Autodesk Inventor part; units mm, degrees
(part 3 of 4)
  line L1419 (-51.1011, -48.3705) -> (-50.3814, -49.0902) construction
  line L1420 (-50.3814, -49.0902) -> (-50.3814, -49.9795) construction
  spline S136 degree 3 poles (-46.3996, -18.0009) (-46.3996, -18.8902) (-47.1193, -19.6113) (-48.0086, -19.6113) knots 0 0 0 0 1 1 1 1
  line L1421 (-46.3996, -18.0009) -> (-46.3996, -18.8902) construction
  line L1422 (-46.3996, -18.8902) -> (-47.1193, -19.6113) construction
  line L1423 (-47.1193, -19.6113) -> (-48.0086, -19.6113) construction
  spline S137 degree 3 poles (-48.0086, -19.6113) (-48.8993, -19.6113) (-49.619, -18.8902) (-49.619, -18.0009) knots 0 0 0 0 1 1 1 1
  line L1424 (-48.0086, -19.6113) -> (-48.8993, -19.6113) construction
  line L1425 (-48.8993, -19.6113) -> (-49.619, -18.8902) construction
  line L1426 (-49.619, -18.8902) -> (-49.619, -18.0009) construction
  spline S138 degree 3 poles (-49.619, -18.0009) (-49.619, -17.1116) (-48.8993, -16.3919) (-48.0086, -16.3919) knots 0 0 0 0 1 1 1 1
  line L1427 (-49.619, -18.0009) -> (-49.619, -17.1116) construction
  line L1428 (-49.619, -17.1116) -> (-48.8993, -16.3919) construction
  line L1429 (-48.8993, -16.3919) -> (-48.0086, -16.3919) construction
  spline S139 degree 3 poles (-48.0086, -16.3919) (-47.1193, -16.3919) (-46.3996, -17.1116) (-46.3996, -18.0009) knots 0 0 0 0 1 1 1 1
  line L1430 (-48.0086, -16.3919) -> (-47.1193, -16.3919) construction
  line L1431 (-47.1193, -16.3919) -> (-46.3996, -17.1116) construction
  line L1432 (-46.3996, -17.1116) -> (-46.3996, -18.0009) construction
  spline S140 degree 3 poles (-72.7019, -7.3708) (-72.7019, -8.0905) (-73.2534, -8.6406) (-73.9731, -8.6406) knots 0 0 0 0 1 1 1 1
  line L1433 (-72.7019, -7.3708) -> (-72.7019, -8.0905) construction
  line L1434 (-72.7019, -8.0905) -> (-73.2534, -8.6406) construction
  line L1435 (-73.2534, -8.6406) -> (-73.9731, -8.6406) construction
  spline S141 degree 3 poles (-73.9731, -8.6406) (-74.6928, -8.6406) (-75.2429, -8.0905) (-75.2429, -7.3708) knots 0 0 0 0 1 1 1 1
  line L1436 (-73.9731, -8.6406) -> (-74.6928, -8.6406) construction
  line L1437 (-74.6928, -8.6406) -> (-75.2429, -8.0905) construction
  line L1438 (-75.2429, -8.0905) -> (-75.2429, -7.3708) construction
  spline S142 degree 3 poles (-75.2429, -7.3708) (-75.2429, -6.6497) (-74.6928, -6.0996) (-73.9731, -6.0996) knots 0 0 0 0 1 1 1 1
  line L1439 (-75.2429, -7.3708) -> (-75.2429, -6.6497) construction
  line L1440 (-75.2429, -6.6497) -> (-74.6928, -6.0996) construction
  line L1441 (-74.6928, -6.0996) -> (-73.9731, -6.0996) construction
  spline S143 degree 3 poles (-73.9731, -6.0996) (-73.2534, -6.0996) (-72.7019, -6.6497) (-72.7019, -7.3708) knots 0 0 0 0 1 1 1 1
  line L1442 (-73.9731, -6.0996) -> (-73.2534, -6.0996) construction
  line L1443 (-73.2534, -6.0996) -> (-72.7019, -6.6497) construction
  line L1444 (-72.7019, -6.6497) -> (-72.7019, -7.3708) construction
  spline S144 degree 3 poles (-72.7019, 7.3694) (-72.7019, 6.6497) (-73.2534, 6.0982) (-73.9731, 6.0982) knots 0 0 0 0 1 1 1 1
  line L1445 (-72.7019, 7.3694) -> (-72.7019, 6.6497) construction
  line L1446 (-72.7019, 6.6497) -> (-73.2534, 6.0982) construction
  line L1447 (-73.2534, 6.0982) -> (-73.9731, 6.0982) construction
  spline S145 degree 3 poles (-73.9731, 6.0982) (-74.6928, 6.0982) (-75.2429, 6.6497) (-75.2429, 7.3694) knots 0 0 0 0 1 1 1 1
  line L1448 (-73.9731, 6.0982) -> (-74.6928, 6.0982) construction
  line L1449 (-74.6928, 6.0982) -> (-75.2429, 6.6497) construction
  line L1450 (-75.2429, 6.6497) -> (-75.2429, 7.3694) construction
  spline S146 degree 3 poles (-75.2429, 7.3694) (-75.2429, 8.0891) (-74.6928, 8.6406) (-73.9731, 8.6406) knots 0 0 0 0 1 1 1 1
  line L1451 (-75.2429, 7.3694) -> (-75.2429, 8.0891) construction
  line L1452 (-75.2429, 8.0891) -> (-74.6928, 8.6406) construction
  line L1453 (-74.6928, 8.6406) -> (-73.9731, 8.6406) construction
  spline S147 degree 3 poles (-73.9731, 8.6406) (-73.2534, 8.6406) (-72.7019, 8.0891) (-72.7019, 7.3694) knots 0 0 0 0 1 1 1 1
  line L1454 (-73.9731, 8.6406) -> (-73.2534, 8.6406) construction
  line L1455 (-73.2534, 8.6406) -> (-72.7019, 8.0891) construction
  line L1456 (-72.7019, 8.0891) -> (-72.7019, 7.3694) construction
  spline S148 degree 3 poles (-46.3996, 18.0009) (-46.3996, 17.1116) (-47.1193, 16.3905) (-48.0086, 16.3905) knots 0 0 0 0 1 1 1 1
  line L1457 (-46.3996, 18.0009) -> (-46.3996, 17.1116) construction
  line L1458 (-46.3996, 17.1116) -> (-47.1193, 16.3905) construction
  line L1459 (-47.1193, 16.3905) -> (-48.0086, 16.3905) construction
  spline S149 degree 3 poles (-48.0086, 16.3905) (-48.8993, 16.3905) (-49.619, 17.1116) (-49.619, 18.0009) knots 0 0 0 0 1 1 1 1
  line L1460 (-48.0086, 16.3905) -> (-48.8993, 16.3905) construction
  line L1461 (-48.8993, 16.3905) -> (-49.619, 17.1116) construction
  line L1462 (-49.619, 17.1116) -> (-49.619, 18.0009) construction
  spline S150 degree 3 poles (-49.619, 18.0009) (-49.619, 18.8902) (-48.8993, 19.6099) (-48.0086, 19.6099) knots 0 0 0 0 1 1 1 1
  line L1463 (-49.619, 18.0009) -> (-49.619, 18.8902) construction
  line L1464 (-49.619, 18.8902) -> (-48.8993, 19.6099) construction
  line L1465 (-48.8993, 19.6099) -> (-48.0086, 19.6099) construction
  spline S151 degree 3 poles (-48.0086, 19.6099) (-47.1193, 19.6099) (-46.3996, 18.8902) (-46.3996, 18.0009) knots 0 0 0 0 1 1 1 1
  line L1466 (-48.0086, 19.6099) -> (-47.1193, 19.6099) construction
  line L1467 (-47.1193, 19.6099) -> (-46.3996, 18.8902) construction
  line L1468 (-46.3996, 18.8902) -> (-46.3996, 18.0009) construction
  spline S152 degree 3 poles (-50.3814, 50.0209) (-50.3814, 49.1316) (-51.1011, 48.4119) (-51.9904, 48.4119) knots 0 0 0 0 1 1 1 1
  line L1469 (-50.3814, 50.0209) -> (-50.3814, 49.1316) construction
  line L1470 (-50.3814, 49.1316) -> (-51.1011, 48.4119) construction
  line L1471 (-51.1011, 48.4119) -> (-51.9904, 48.4119) construction
  spline S153 degree 3 poles (-51.9904, 48.4119) (-52.8797, 48.4119) (-53.6008, 49.1316) (-53.6008, 50.0209) knots 0 0 0 0 1 1 1 1
  line L1472 (-51.9904, 48.4119) -> (-52.8797, 48.4119) construction
  line L1473 (-52.8797, 48.4119) -> (-53.6008, 49.1316) construction
  line L1474 (-53.6008, 49.1316) -> (-53.6008, 50.0209) construction
  spline S154 degree 3 poles (-53.6008, 50.0209) (-53.6008, 50.9102) (-52.8797, 51.6299) (-51.9904, 51.6299) knots 0 0 0 0 1 1 1 1
  line L1475 (-53.6008, 50.0209) -> (-53.6008, 50.9102) construction
  line L1476 (-53.6008, 50.9102) -> (-52.8797, 51.6299) construction
  line L1477 (-52.8797, 51.6299) -> (-51.9904, 51.6299) construction
  spline S155 degree 3 poles (-51.9904, 51.6299) (-51.1011, 51.6299) (-50.3814, 50.9102) (-50.3814, 50.0209) knots 0 0 0 0 1 1 1 1
  line L1478 (-51.9904, 51.6299) -> (-51.1011, 51.6299) construction
  line L1479 (-51.1011, 51.6299) -> (-50.3814, 50.9102) construction
  line L1480 (-50.3814, 50.9102) -> (-50.3814, 50.0209) construction
  spline S156 degree 3 poles (-7.7299, 44.0068) (-7.7299, 43.2871) (-8.2801, 42.7356) (-8.9998, 42.7356) knots 0 0 0 0 1 1 1 1
  line L1481 (-7.7299, 44.0068) -> (-7.7299, 43.2871) construction
  line L1482 (-7.7299, 43.2871) -> (-8.2801, 42.7356) construction
  line L1483 (-8.2801, 42.7356) -> (-8.9998, 42.7356) construction
  spline S157 degree 3 poles (-8.9998, 42.7356) (-9.7208, 42.7356) (-10.271, 43.2871) (-10.271, 44.0068) knots 0 0 0 0 1 1 1 1
  line L1484 (-8.9998, 42.7356) -> (-9.7208, 42.7356) construction
  line L1485 (-9.7208, 42.7356) -> (-10.271, 43.2871) construction
  line L1486 (-10.271, 43.2871) -> (-10.271, 44.0068) construction
  spline S158 degree 3 poles (-10.271, 44.0068) (-10.271, 44.7265) (-9.7208, 45.2766) (-8.9998, 45.2766) knots 0 0 0 0 1 1 1 1
  line L1487 (-10.271, 44.0068) -> (-10.271, 44.7265) construction
  line L1488 (-10.271, 44.7265) -> (-9.7208, 45.2766) construction
  line L1489 (-9.7208, 45.2766) -> (-8.9998, 45.2766) construction
  spline S159 degree 3 poles (-8.9998, 45.2766) (-8.2801, 45.2766) (-7.7299, 44.7265) (-7.7299, 44.0068) knots 0 0 0 0 1 1 1 1
  line L1490 (-8.9998, 45.2766) -> (-8.2801, 45.2766) construction
  line L1491 (-8.2801, 45.2766) -> (-7.7299, 44.7265) construction
  line L1492 (-7.7299, 44.7265) -> (-7.7299, 44.0068) construction
  spline S160 degree 3 poles (52.626, 50.0209) (52.626, 49.1316) (51.9063, 48.4119) (51.017, 48.4119) knots 0 0 0 0 1 1 1 1
  line L1493 (52.626, 50.0209) -> (52.626, 49.1316) construction
  line L1494 (52.626, 49.1316) -> (51.9063, 48.4119) construction
  line L1495 (51.9063, 48.4119) -> (51.017, 48.4119) construction
  spline S161 degree 3 poles (51.017, 48.4119) (50.1277, 48.4119) (49.408, 49.1316) (49.408, 50.0209) knots 0 0 0 0 1 1 1 1
  line L1496 (51.017, 48.4119) -> (50.1277, 48.4119) construction
  line L1497 (50.1277, 48.4119) -> (49.408, 49.1316) construction
  line L1498 (49.408, 49.1316) -> (49.408, 50.0209) construction
  spline S162 degree 3 poles (49.408, 50.0209) (49.408, 50.9102) (50.1277, 51.6299) (51.017, 51.6299) knots 0 0 0 0 1 1 1 1
  line L1499 (49.408, 50.0209) -> (49.408, 50.9102) construction
  line L1500 (49.408, 50.9102) -> (50.1277, 51.6299) construction
  line L1501 (50.1277, 51.6299) -> (51.017, 51.6299) construction
  spline S163 degree 3 poles (51.017, 51.6299) (51.9063, 51.6299) (52.626, 50.9102) (52.626, 50.0209) knots 0 0 0 0 1 1 1 1
  line L1502 (51.017, 51.6299) -> (51.9063, 51.6299) construction
  line L1503 (51.9063, 51.6299) -> (52.626, 50.9102) construction
  line L1504 (52.626, 50.9102) -> (52.626, 50.0209) construction
  spline S164 degree 3 poles (10.271, 44.0068) (10.271, 43.2871) (9.7208, 42.7356) (9.0011, 42.7356) knots 0 0 0 0 1 1 1 1
  line L1505 (10.271, 44.0068) -> (10.271, 43.2871) construction
  line L1506 (10.271, 43.2871) -> (9.7208, 42.7356) construction
  line L1507 (9.7208, 42.7356) -> (9.0011, 42.7356) construction
  spline S165 degree 3 poles (9.0011, 42.7356) (8.28, 42.7356) (7.7299, 43.2871) (7.7299, 44.0068) knots 0 0 0 0 1 1 1 1
  line L1508 (9.0011, 42.7356) -> (8.28, 42.7356) construction
  line L1509 (8.28, 42.7356) -> (7.7299, 43.2871) construction
  line L1510 (7.7299, 43.2871) -> (7.7299, 44.0068) construction
  spline S166 degree 3 poles (7.7299, 44.0068) (7.7299, 44.7265) (8.28, 45.2766) (9.0011, 45.2766) knots 0 0 0 0 1 1 1 1
  line L1511 (7.7299, 44.0068) -> (7.7299, 44.7265) construction
  line L1512 (7.7299, 44.7265) -> (8.28, 45.2766) construction
  line L1513 (8.28, 45.2766) -> (9.0011, 45.2766) construction
  spline S167 degree 3 poles (9.0011, 45.2766) (9.7208, 45.2766) (10.271, 44.7265) (10.271, 44.0068) knots 0 0 0 0 1 1 1 1
  line L1514 (9.0011, 45.2766) -> (9.7208, 45.2766) construction
  line L1515 (9.7208, 45.2766) -> (10.271, 44.7265) construction
  line L1516 (10.271, 44.7265) -> (10.271, 44.0068) construction
  spline S168 degree 3 poles (20.606, 18.0009) (20.606, 17.1116) (19.8863, 16.3905) (18.997, 16.3905) knots 0 0 0 0 1 1 1 1
  line L1517 (20.606, 18.0009) -> (20.606, 17.1116) construction
  line L1518 (20.606, 17.1116) -> (19.8863, 16.3905) construction
  line L1519 (19.8863, 16.3905) -> (18.997, 16.3905) construction
  spline S169 degree 3 poles (18.997, 16.3905) (18.1064, 16.3905) (17.3867, 17.1116) (17.3867, 18.0009) knots 0 0 0 0 1 1 1 1
  line L1520 (18.997, 16.3905) -> (18.1064, 16.3905) construction
  line L1521 (18.1064, 16.3905) -> (17.3867, 17.1116) construction
  line L1522 (17.3867, 17.1116) -> (17.3867, 18.0009) construction
  spline S170 degree 3 poles (17.3867, 18.0009) (17.3867, 18.8902) (18.1064, 19.6099) (18.997, 19.6099) knots 0 0 0 0 1 1 1 1
  line L1523 (17.3867, 18.0009) -> (17.3867, 18.8902) construction
  line L1524 (17.3867, 18.8902) -> (18.1064, 19.6099) construction
  line L1525 (18.1064, 19.6099) -> (18.997, 19.6099) construction
  spline S171 degree 3 poles (18.997, 19.6099) (19.8863, 19.6099) (20.606, 18.8902) (20.606, 18.0009) knots 0 0 0 0 1 1 1 1
  line L1526 (18.997, 19.6099) -> (19.8863, 19.6099) construction
  line L1527 (19.8863, 19.6099) -> (20.606, 18.8902) construction
  line L1528 (20.606, 18.8902) -> (20.606, 18.0009) construction
  spline S172 degree 3 poles (20.606, -18.0009) (20.606, -18.8902) (19.8863, -19.6113) (18.997, -19.6113) knots 0 0 0 0 1 1 1 1
  line L1529 (20.606, -18.0009) -> (20.606, -18.8902) construction
  line L1530 (20.606, -18.8902) -> (19.8863, -19.6113) construction
  line L1531 (19.8863, -19.6113) -> (18.997, -19.6113) construction
  spline S173 degree 3 poles (18.997, -19.6113) (18.1064, -19.6113) (17.3867, -18.8902) (17.3867, -18.0009) knots 0 0 0 0 1 1 1 1
  line L1532 (18.997, -19.6113) -> (18.1064, -19.6113) construction
  line L1533 (18.1064, -19.6113) -> (17.3867, -18.8902) construction
  line L1534 (17.3867, -18.8902) -> (17.3867, -18.0009) construction
  spline S174 degree 3 poles (17.3867, -18.0009) (17.3867, -17.1116) (18.1064, -16.3919) (18.997, -16.3919) knots 0 0 0 0 1 1 1 1
  line L1535 (17.3867, -18.0009) -> (17.3867, -17.1116) construction
  line L1536 (17.3867, -17.1116) -> (18.1064, -16.3919) construction
  line L1537 (18.1064, -16.3919) -> (18.997, -16.3919) construction
  spline S175 degree 3 poles (18.997, -16.3919) (19.8863, -16.3919) (20.606, -17.1116) (20.606, -18.0009) knots 0 0 0 0 1 1 1 1
  line L1538 (18.997, -16.3919) -> (19.8863, -16.3919) construction
  line L1539 (19.8863, -16.3919) -> (20.606, -17.1116) construction
  line L1540 (20.606, -17.1116) -> (20.606, -18.0009) construction
  spline S176 degree 3 poles (52.626, -49.9795) (52.626, -50.8688) (51.9063, -51.5885) (51.017, -51.5885) knots 0 0 0 0 1 1 1 1
  line L1541 (52.626, -49.9795) -> (52.626, -50.8688) construction
  line L1542 (52.626, -50.8688) -> (51.9063, -51.5885) construction
  line L1543 (51.9063, -51.5885) -> (51.017, -51.5885) construction
  spline S177 degree 3 poles (51.017, -51.5885) (50.1277, -51.5885) (49.408, -50.8688) (49.408, -49.9795) knots 0 0 0 0 1 1 1 1
  line L1544 (51.017, -51.5885) -> (50.1277, -51.5885) construction
  line L1545 (50.1277, -51.5885) -> (49.408, -50.8688) construction
  line L1546 (49.408, -50.8688) -> (49.408, -49.9795) construction
  spline S178 degree 3 poles (49.408, -49.9795) (49.408, -49.0902) (50.1277, -48.3705) (51.017, -48.3705) knots 0 0 0 0 1 1 1 1
  line L1547 (49.408, -49.9795) -> (49.408, -49.0902) construction
  line L1548 (49.408, -49.0902) -> (50.1277, -48.3705) construction
  line L1549 (50.1277, -48.3705) -> (51.017, -48.3705) construction
  spline S179 degree 3 poles (51.017, -48.3705) (51.9063, -48.3705) (52.626, -49.0902) (52.626, -49.9795) knots 0 0 0 0 1 1 1 1
  line L1550 (51.017, -48.3705) -> (51.9063, -48.3705) construction
  line L1551 (51.9063, -48.3705) -> (52.626, -49.0902) construction
  line L1552 (52.626, -49.0902) -> (52.626, -49.9795) construction
  spline S180 degree 3 poles (68.2982, 7.3694) (68.2982, 6.6497) (67.7467, 6.0982) (67.027, 6.0982) knots 0 0 0 0 1 1 1 1
  line L1553 (68.2982, 7.3694) -> (68.2982, 6.6497) construction
  line L1554 (68.2982, 6.6497) -> (67.7467, 6.0982) construction
  line L1555 (67.7467, 6.0982) -> (67.027, 6.0982) construction
  spline S181 degree 3 poles (67.027, 6.0982) (66.3073, 6.0982) (65.7558, 6.6497) (65.7558, 7.3694) knots 0 0 0 0 1 1 1 1
  line L1556 (67.027, 6.0982) -> (66.3073, 6.0982) construction
  line L1557 (66.3073, 6.0982) -> (65.7558, 6.6497) construction
  line L1558 (65.7558, 6.6497) -> (65.7558, 7.3694) construction
  spline S182 degree 3 poles (65.7558, 7.3694) (65.7558, 8.0891) (66.3073, 8.6406) (67.027, 8.6406) knots 0 0 0 0 1 1 1 1
  line L1559 (65.7558, 7.3694) -> (65.7558, 8.0891) construction
  line L1560 (65.7558, 8.0891) -> (66.3073, 8.6406) construction
  line L1561 (66.3073, 8.6406) -> (67.027, 8.6406) construction
  spline S183 degree 3 poles (67.027, 8.6406) (67.7467, 8.6406) (68.2982, 8.0891) (68.2982, 7.3694) knots 0 0 0 0 1 1 1 1
  line L1562 (67.027, 8.6406) -> (67.7467, 8.6406) construction
  line L1563 (67.7467, 8.6406) -> (68.2982, 8.0891) construction
  line L1564 (68.2982, 8.0891) -> (68.2982, 7.3694) construction
  spline S184 degree 3 poles (68.2982, -7.3708) (68.2982, -8.0905) (67.7467, -8.6406) (67.027, -8.6406) knots 0 0 0 0 1 1 1 1
  line L1565 (68.2982, -7.3708) -> (68.2982, -8.0905) construction
  line L1566 (68.2982, -8.0905) -> (67.7467, -8.6406) construction
  line L1567 (67.7467, -8.6406) -> (67.027, -8.6406) construction
  spline S185 degree 3 poles (67.027, -8.6406) (66.3073, -8.6406) (65.7558, -8.0905) (65.7558, -7.3708) knots 0 0 0 0 1 1 1 1
  line L1568 (67.027, -8.6406) -> (66.3073, -8.6406) construction
  line L1569 (66.3073, -8.6406) -> (65.7558, -8.0905) construction
  line L1570 (65.7558, -8.0905) -> (65.7558, -7.3708) construction
  spline S186 degree 3 poles (65.7558, -7.3708) (65.7558, -6.6497) (66.3073, -6.0996) (67.027, -6.0996) knots 0 0 0 0 1 1 1 1
  line L1571 (65.7558, -7.3708) -> (65.7558, -6.6497) construction
  line L1572 (65.7558, -6.6497) -> (66.3073, -6.0996) construction
  line L1573 (66.3073, -6.0996) -> (67.027, -6.0996) construction
  spline S187 degree 3 poles (67.027, -6.0996) (67.7467, -6.0996) (68.2982, -6.6497) (68.2982, -7.3708) knots 0 0 0 0 1 1 1 1
  line L1574 (67.027, -6.0996) -> (67.7467, -6.0996) construction
  line L1575 (67.7467, -6.0996) -> (68.2982, -6.6497) construction
  line L1576 (68.2982, -6.6497) -> (68.2982, -7.3708) construction
  spline S188 degree 3 poles (-25.3917, 18.0009) (-25.3917, 17.1116) (-26.1114, 16.3905) (-27.0006, 16.3905) knots 0 0 0 0 1 1 1 1
  line L1577 (-25.3917, 18.0009) -> (-25.3917, 17.1116) construction
  line L1578 (-25.3917, 17.1116) -> (-26.1114, 16.3905) construction
  line L1579 (-26.1114, 16.3905) -> (-27.0006, 16.3905) construction
  spline S189 degree 3 poles (-27.0006, 16.3905) (-27.8899, 16.3905) (-28.611, 17.1116) (-28.611, 18.0009) knots 0 0 0 0 1 1 1 1
  line L1580 (-27.0006, 16.3905) -> (-27.8899, 16.3905) construction
  line L1581 (-27.8899, 16.3905) -> (-28.611, 17.1116) construction
  line L1582 (-28.611, 17.1116) -> (-28.611, 18.0009) construction
  spline S190 degree 3 poles (-28.611, 18.0009) (-28.611, 18.8902) (-27.8899, 19.6099) (-27.0006, 19.6099) knots 0 0 0 0 1 1 1 1
  line L1583 (-28.611, 18.0009) -> (-28.611, 18.8902) construction
  line L1584 (-28.611, 18.8902) -> (-27.8899, 19.6099) construction
  line L1585 (-27.8899, 19.6099) -> (-27.0006, 19.6099) construction
  spline S191 degree 3 poles (-27.0006, 19.6099) (-26.1114, 19.6099) (-25.3917, 18.8902) (-25.3917, 18.0009) knots 0 0 0 0 1 1 1 1
  line L1586 (-27.0006, 19.6099) -> (-26.1114, 19.6099) construction
  line L1587 (-26.1114, 19.6099) -> (-25.3917, 18.8902) construction
  line L1588 (-25.3917, 18.8902) -> (-25.3917, 18.0009) construction
  spline S192 degree 3 poles (-25.3917, -18.0009) (-25.3917, -18.8902) (-26.1114, -19.6113) (-27.0006, -19.6113) knots 0 0 0 0 1 1 1 1
  line L1589 (-25.3917, -18.0009) -> (-25.3917, -18.8902) construction
  line L1590 (-25.3917, -18.8902) -> (-26.1114, -19.6113) construction
  line L1591 (-26.1114, -19.6113) -> (-27.0006, -19.6113) construction
  spline S193 degree 3 poles (-27.0006, -19.6113) (-27.8899, -19.6113) (-28.611, -18.8902) (-28.611, -18.0009) knots 0 0 0 0 1 1 1 1
  line L1592 (-27.0006, -19.6113) -> (-27.8899, -19.6113) construction
  line L1593 (-27.8899, -19.6113) -> (-28.611, -18.8902) construction
  line L1594 (-28.611, -18.8902) -> (-28.611, -18.0009) construction
  spline S194 degree 3 poles (-28.611, -18.0009) (-28.611, -17.1116) (-27.8899, -16.3919) (-27.0006, -16.3919) knots 0 0 0 0 1 1 1 1
  line L1595 (-28.611, -18.0009) -> (-28.611, -17.1116) construction
  line L1596 (-28.611, -17.1116) -> (-27.8899, -16.3919) construction
  line L1597 (-27.8899, -16.3919) -> (-27.0006, -16.3919) construction
  spline S195 degree 3 poles (-27.0006, -16.3919) (-26.1114, -16.3919) (-25.3917, -17.1116) (-25.3917, -18.0009) knots 0 0 0 0 1 1 1 1
  line L1598 (-27.0006, -16.3919) -> (-26.1114, -16.3919) construction
  line L1599 (-26.1114, -16.3919) -> (-25.3917, -17.1116) construction
  line L1600 (-25.3917, -17.1116) -> (-25.3917, -18.0009) construction
  line L1601 (-33.9895, 68.0217) -> (-25.0111, 68.0217)
  line L1602 (-25.0111, 50.0209) -> (-6.5015, 50.0209)
  line L1603 (6.5015, 50.0209) -> (25.0111, 50.0209)
  line L1604 (-6.5015, 50.0209) -> (-6.5015, 60.0168)
  line L1605 (-6.5015, 60.0168) -> (6.5015, 60.0168)
  line L1606 (6.5015, 60.0168) -> (6.5015, 50.0209)
  line L1607 (-25.0111, -67.9804) -> (-33.9895, -67.9804)
  line L1608 (-6.5015, -59.9754) -> (6.5015, -59.9754)
  line L1609 (6.5015, -59.9754) -> (6.5015, -49.9795)
  line L1610 (6.5015, -49.9795) -> (25.0111, -49.9795)
  line L1611 (-25.0111, -49.9795) -> (-6.5015, -49.9795)
  line L1612 (-6.5015, -49.9795) -> (-6.5015, -59.9754)
  line L1613 (-33.9895, 68.0217) -> (-36.9965, 66.4541)
  line L1614 (-36.9965, 66.4541) -> (-39.9195, 64.7183)
  line L1615 (-39.9195, 64.7183) -> (-42.7569, 62.897)
  line L1616 (-42.7569, 62.897) -> (-45.5103, 60.9488)
  line L1617 (-45.5103, 60.9488) -> (-48.1782, 58.8738)
  line L1618 (-48.1782, 58.8738) -> (-50.7206, 56.6705)
  line L1619 (-50.7206, 56.6705) -> (-53.2189, 54.3405)
  line L1620 (-53.2189, 54.3405) -> (-55.5903, 51.9263)
  line L1621 (-55.5903, 51.9263) -> (-57.8363, 49.428)
  line L1622 (-57.8363, 49.428) -> (-59.954, 46.8015)
  line L1623 (-59.954, 46.8015) -> (-61.9863, 44.0909)
  line L1624 (-61.9863, 44.0909) -> (-63.8917, 41.2962)
  line L1625 (-63.8917, 41.2962) -> (-65.6289, 38.3732)
  line L1626 (-65.6289, 38.3732) -> (-67.2807, 35.4503)
  line L1627 (-67.2807, 35.4503) -> (-68.7628, 32.4019)
  line L1628 (-68.7628, 32.4019) -> (-70.1609, 29.3094)
  line L1629 (-70.1609, 29.3094) -> (-71.3893, 26.1755)
  line L1630 (-71.3893, 26.1755) -> (-72.4482, 22.9561)
  line L1631 (-72.4482, 22.9561) -> (-73.3802, 19.6954)
  line L1632 (-73.3802, 19.6954) -> (-74.9892, 18.5083)
  line L1633 (-74.9892, 18.5083) -> (-76.4714, 17.153)
  line L1634 (-76.4714, 17.153) -> (-77.8267, 15.6708)
  line L1635 (-77.8267, 15.6708) -> (-79.0979, 14.1032)
  line L1636 (-79.0979, 14.1032) -> (-80.1995, 12.4101)
  line L1637 (-80.1995, 12.4101) -> (-81.1729, 10.6729)
  line L1638 (-81.1729, 10.6729) -> (-81.9781, 8.8515)
  line L1639 (-81.9781, 8.8515) -> (-82.6137, 6.9461)
  line L1640 (-82.6137, 6.9461) -> (-83.1211, 4.9979)
  line L1641 (-83.1211, 4.9979) -> (-83.4603, 3.007)
  line L1642 (-83.4603, 3.007) -> (-83.6298, 1.0161)
  line L1643 (-83.6298, 1.0161) -> (-83.6298, -0.9748)
  line L1644 (-83.6298, -0.9748) -> (-83.4603, -3.007)
  line L1645 (-83.4603, -3.007) -> (-83.1211, -4.9566)
  line L1646 (-83.1211, -4.9566) -> (-82.6137, -6.9048)
  line L1647 (-82.6137, -6.9048) -> (-81.9781, -8.8102)
  line L1648 (-81.9781, -8.8102) -> (-81.1729, -10.6315)
  line L1649 (-81.1729, -10.6315) -> (-80.1995, -12.4101)
  line L1650 (-80.1995, -12.4101) -> (-79.0979, -14.0618)
  line L1651 (-79.0979, -14.0618) -> (-77.8267, -15.6722)
  line L1652 (-77.8267, -15.6722) -> (-76.4714, -17.1116)
  line L1653 (-76.4714, -17.1116) -> (-74.9892, -18.4669)
  line L1654 (-74.9892, -18.4669) -> (-73.3802, -19.6954)
  line L1655 (-73.3802, -19.6954) -> (-72.4482, -22.9147)
  line L1656 (-72.4482, -22.9147) -> (-71.3466, -26.1341)
  line L1657 (-71.3466, -26.1341) -> (-70.1181, -29.268)
  line L1658 (-70.1181, -29.268) -> (-68.7628, -32.3591)
  line L1659 (-68.7628, -32.3591) -> (-67.2379, -35.4089)
  line L1660 (-67.2379, -35.4089) -> (-65.5862, -38.3319)
  line L1661 (-65.5862, -38.3319) -> (-63.8504, -41.2121)
  line L1662 (-63.8504, -41.2121) -> (-61.9436, -44.0068)
  line L1663 (-61.9436, -44.0068) -> (-59.9113, -46.7174)
  line L1664 (-59.9113, -46.7174) -> (-57.7935, -49.3439)
  line L1665 (-57.7935, -49.3439) -> (-55.5489, -51.8849)
  line L1666 (-55.5489, -51.8849) -> (-53.1761, -54.2991)
  line L1667 (-53.1761, -54.2991) -> (-50.7206, -56.5864)
  line L1668 (-50.7206, -56.5864) -> (-48.1368, -58.7897)
  line L1669 (-48.1368, -58.7897) -> (-45.4676, -60.9074)
  line L1670 (-45.4676, -60.9074) -> (-42.7142, -62.8556)
  line L1671 (-42.7142, -62.8556) -> (-39.8767, -64.6769)
  line L1672 (-39.8767, -64.6769) -> (-36.9965, -66.4128)
  line L1673 (-36.9965, -66.4128) -> (-33.9895, -67.9804)
  line L1674 (34.0322, -67.9804) -> (37.1248, -66.3287)
  line L1675 (37.1248, -66.3287) -> (40.1318, -64.5501)
  line L1676 (40.1318, -64.5501) -> (43.0547, -62.6433)
  line L1677 (43.0547, -62.6433) -> (45.9336, -60.611)
  line L1678 (45.9336, -60.611) -> (48.6456, -58.4078)
  line L1679 (48.6456, -58.4078) -> (51.3134, -56.1204)
  line L1680 (51.3134, -56.1204) -> (53.8545, -53.6649)
  line L1681 (53.8545, -53.6649) -> (56.2686, -51.1225)
  line L1682 (56.2686, -51.1225) -> (58.556, -48.4974)
  line L1683 (58.556, -48.4974) -> (60.7165, -45.744)
  line L1684 (60.7165, -45.744) -> (62.7915, -42.9065)
  line L1685 (62.7915, -42.9065) -> (64.6969, -39.9409)
  line L1686 (64.6969, -39.9409) -> (66.4769, -36.9338)
  line L1687 (66.4769, -36.9338) -> (68.0859, -33.8427)
  line L1688 (68.0859, -33.8427) -> (69.568, -30.666)
  line L1689 (69.568, -30.666) -> (70.9233, -27.4039)
  line L1690 (70.9233, -27.4039) -> (72.109, -24.1005)
  line L1691 (72.109, -24.1005) -> (73.1679, -20.7542)
  line L1692 (73.1679, -20.7542) -> (74.0158, -17.3653)
  line L1693 (74.0158, -17.3653) -> (74.7355, -13.935)
  line L1694 (74.7355, -13.935) -> (75.3284, -10.4619)
  line L1695 (75.3284, -10.4619) -> (75.7103, -6.9889)
  line L1696 (75.7103, -6.9889) -> (75.964, -3.5158)
  line L1697 (75.964, -3.5158) -> (76.0481, 0)
  line L1698 (76.0481, 0) -> (75.964, 3.5144)
  line L1699 (75.964, 3.5144) -> (75.7103, 7.0302)
  line L1700 (75.7103, 7.0302) -> (75.3284, 10.5033)
  line L1701 (75.3284, 10.5033) -> (74.7355, 13.9763)
  line L1702 (74.7355, 13.9763) -> (74.0158, 17.408)
  line L1703 (74.0158, 17.408) -> (73.1679, 20.7956)
  line L1704 (73.1679, 20.7956) -> (72.109, 24.1418)
  line L1705 (72.109, 24.1418) -> (70.9233, 27.4453)
  line L1706 (70.9233, 27.4453) -> (69.568, 30.6647)
  line L1707 (69.568, 30.6647) -> (68.0859, 33.8413)
  line L1708 (68.0859, 33.8413) -> (66.4769, 36.9338)
  line L1709 (66.4769, 36.9338) -> (64.6969, 39.9822)
  line L1710 (64.6969, 39.9822) -> (62.7915, 42.9052)
  line L1711 (62.7915, 42.9052) -> (60.7165, 45.7854)
  line L1712 (60.7165, 45.7854) -> (58.556, 48.496)
  line L1713 (58.556, 48.496) -> (56.2686, 51.1638)
  line L1714 (56.2686, 51.1638) -> (53.8545, 53.7062)
  line L1715 (53.8545, 53.7062) -> (51.3134, 56.1204)
  line L1716 (51.3134, 56.1204) -> (48.6456, 58.4491)
  line L1717 (48.6456, 58.4491) -> (45.9336, 60.6096)
  line L1718 (45.9336, 60.6096) -> (43.0547, 62.6846)
  line L1719 (43.0547, 62.6846) -> (40.1318, 64.5914)
  line L1720 (40.1318, 64.5914) -> (37.1248, 66.37)
  line L1721 (37.1248, 66.37) -> (34.0322, 68.0217)
  line L1722 (-25.0111, 50.0209) -> (-25.0111, 68.0217)
  line L1723 (25.0111, 50.0209) -> (25.0111, 68.0217)
  line L1724 (25.0111, 68.0217) -> (34.0322, 68.0217)
  line L1725 (-25.0111, -67.9804) -> (-25.0111, -49.9795)
  line L1726 (25.0111, -49.9795) -> (25.0111, -67.9804)
  line L1727 (25.0111, -67.9804) -> (34.0322, -67.9804)
  line L1728 (76.0481, 0) -> (-83.6298, 0)
  line L1729 (0, -67.9804) -> (0, 68.0217)
  point P0 (0, 0)
  point P1 (0, 0)
  point P2 (0, 0)
  point P3 (51.017, 50.0209)
  point P4 (51.017, -49.9795)
  point P5 (18.997, -18.0009)
  point P6 (18.997, 18.0009)
  point P7 (9.0011, 44.0068)
  point P8 (10.271, -44.0068)
  point P9 (9.0011, -44.0068)
  point P10 (-8.9998, 44.0068)
  point P11 (-8.9998, -44.0068)
  point P12 (67.027, 7.3694)
  point P13 (67.027, -7.3708)
  point P14 (-51.9904, 48.4119)
  point P15 (-50.3814, 50.0209)
  point P16 (-51.9904, 50.0209)
  point P17 (-46.3996, 18.0009)
  point P18 (-48.0086, 16.3905)
  point P19 (-48.0086, 18.0009)
  point P20 (-27.0006, 18.0009)
  point P21 (41.0211, 40.025)
  point P22 (-31.9986, 40.025)
  point P23 (-53.9813, 4.9979)
  constraints: 2284 end point, 30 coincident, 4 point on line, 1 perpendicular, 588 other
sketch "Sketch4" plane through (0, 0, 0) normal (0, 1, 0) x (-1, 0, 0)
  line L0 (51.017, 48.4097) -> (50.1277, 48.4097) construction
  spline S0 degree 3 poles (51.017, 48.4097) (50.1277, 48.4097) (49.408, 49.1311) (49.408, 50.0209) knots 0 0 0 0 1 1 1 1
  line L1 (50.1277, 48.4097) -> (49.408, 49.1311) construction
  line L2 (49.408, 49.1311) -> (49.408, 50.0209) construction
  line L3 (52.626, 49.1311) -> (51.9063, 48.4097) construction
  spline S1 degree 3 poles (52.626, 50.0209) (52.626, 49.1311) (51.9063, 48.4097) (51.017, 48.4097) knots 0 0 0 0 1 1 1 1
  line L4 (52.626, 50.0209) -> (52.626, 49.1311) construction
  line L5 (51.9063, 48.4097) -> (51.017, 48.4097) construction
  line L6 (51.017, 50.0209) -> (48.167, 50.0209)
  line L7 (50.1277, 51.6306) -> (51.017, 51.6306) construction
  spline S2 degree 3 poles (49.408, 50.0209) (49.408, 50.9106) (50.1277, 51.6306) (51.017, 51.6306) knots 0 0 0 0 1 1 1 1
  line L8 (49.408, 50.0209) -> (49.408, 50.9106) construction
  line L9 (49.408, 50.9106) -> (50.1277, 51.6306) construction
  line L10 (53.867, 48.3754) -> (51.017, 50.0209)
  line L11 (48.167, 48.3754) -> (48.167, 51.6663)
  line L12 (53.867, 51.6663) -> (53.867, 48.3754)
  circle A0 centre (53.617, 51.522) radius 0.5
  line L13 (53.617, 47.9424) -> (47.917, 51.2333)
  line L14 (48.417, 52.0993) -> (53.617, 47.9424) construction
  line L15 (48.417, 52.0993) -> (54.117, 48.8084)
  line L16 (54.117, 48.8084) -> (47.917, 51.2333) construction
  circle A1 centre (51.017, 50.0209) radius 2.5
  circle A2 centre (48.417, 51.522) radius 0.5
  line L17 (47.917, 51.2333) -> (48.417, 52.0993)
  line L18 (48.167, 51.6663) -> (51.017, 53.3118)
  circle A3 centre (48.417, 48.5197) radius 0.5
  line L19 (51.017, 46.73) -> (48.167, 48.3754)
  circle A4 centre (51.017, 47.0186) radius 0.5
  line L20 (53.367, 48.0867) -> (53.867, 48.9528)
  circle A5 centre (53.617, 48.5197) radius 0.5
  line L21 (53.867, 48.3754) -> (51.017, 46.73)
  line L22 (54.117, 48.8084) -> (53.617, 47.9424)
  circle A6 centre (51.017, 53.0231) radius 0.5
  line L23 (51.017, 51.6306) -> (51.9063, 51.6306) construction
  spline S3 degree 3 poles (51.017, 51.6306) (51.9063, 51.6306) (52.626, 50.9106) (52.626, 50.0209) knots 0 0 0 0 1 1 1 1
  line L24 (51.9063, 51.6306) -> (52.626, 50.9106) construction
  line L25 (52.626, 50.9106) -> (52.626, 50.0209) construction
  line L26 (51.017, 53.3118) -> (53.867, 51.6663)
  line L27 (18.9583, 16.4287) -> (18.069, 16.4287) construction
  spline S4 degree 3 poles (18.9583, 16.4287) (18.069, 16.4287) (17.3493, 17.1502) (17.3493, 18.0399) knots 0 0 0 0 1 1 1 1
  line L28 (18.069, 16.4287) -> (17.3493, 17.1502) construction
  line L29 (17.3493, 17.1502) -> (17.3493, 18.0399) construction
  circle A7 centre (21.5583, 19.541) radius 0.5
  line L30 (17.3493, 18.0399) -> (17.3493, 18.9296) construction
  spline S5 degree 3 poles (17.3493, 18.0399) (17.3493, 18.9296) (18.069, 19.6497) (18.9583, 19.6497) knots 0 0 0 0 1 1 1 1
  line L31 (17.3493, 18.9296) -> (18.069, 19.6497) construction
  line L32 (18.069, 19.6497) -> (18.9583, 19.6497) construction
  line L33 (19.8475, 16.4287) -> (18.9583, 16.4287) construction
  spline S6 degree 3 poles (20.5672, 18.0399) (20.5672, 17.1502) (19.8475, 16.4287) (18.9583, 16.4287) knots 0 0 0 0 1 1 1 1
  line L34 (20.5672, 18.0399) -> (20.5672, 17.1502) construction
  line L35 (20.5672, 17.1502) -> (19.8475, 16.4287) construction
  line L36 (18.9583, 19.6497) -> (19.8475, 19.6497) construction
  spline S7 degree 3 poles (18.9583, 19.6497) (19.8475, 19.6497) (20.5672, 18.9296) (20.5672, 18.0399) knots 0 0 0 0 1 1 1 1
  line L37 (19.8475, 19.6497) -> (20.5672, 18.9296) construction
  line L38 (20.5672, 18.9296) -> (20.5672, 18.0399) construction
  line L39 (21.5583, 15.9614) -> (15.8583, 19.2523)
  line L40 (16.3583, 20.1183) -> (21.5583, 15.9614) construction
  circle A8 centre (18.9583, 18.0399) radius 2.5
  line L41 (16.3583, 20.1183) -> (22.0583, 16.8274)
  line L42 (21.8083, 16.3944) -> (18.9583, 18.0399)
  line L43 (18.9583, 21.3308) -> (21.8083, 19.6853)
  line L44 (21.8083, 19.6853) -> (21.8083, 16.3944)
  line L45 (18.9583, 18.0399) -> (16.1083, 18.0399)
  circle A9 centre (18.9583, 21.0421) radius 0.5
  line L46 (16.1083, 19.6853) -> (18.9583, 21.3308)
  circle A10 centre (16.3583, 16.5388) radius 0.5
  line L47 (18.9583, 14.749) -> (16.1083, 16.3944)
  circle A11 centre (16.3583, 19.541) radius 0.5
  line L48 (15.8583, 19.2523) -> (16.3583, 20.1183)
  line L49 (16.1083, 16.3944) -> (16.1083, 19.6853)
  line L50 (22.0583, 16.8274) -> (15.8583, 19.2523) construction
  circle A12 centre (18.9583, 15.0377) radius 0.5
  line L51 (21.3083, 16.1058) -> (21.8083, 16.9718)
  line L52 (21.8083, 16.3944) -> (18.9583, 14.749)
  circle A13 centre (21.5583, 16.5388) radius 0.5
  line L53 (22.0583, 16.8274) -> (21.5583, 15.9614)
  line L54 (-27.0006, 16.3897) -> (-27.8899, 16.3897) construction
  spline S8 degree 3 poles (-27.0006, 16.3897) (-27.8899, 16.3897) (-28.6096, 17.1112) (-28.6096, 18.0009) knots 0 0 0 0 1 1 1 1
  line L55 (-27.8899, 16.3897) -> (-28.6096, 17.1112) construction
  line L56 (-28.6096, 17.1112) -> (-28.6096, 18.0009) construction
  circle A14 centre (-24.4006, 19.502) radius 0.5
  line L57 (-28.6096, 18.0009) -> (-28.6096, 18.8906) construction
  spline S9 degree 3 poles (-28.6096, 18.0009) (-28.6096, 18.8906) (-27.8899, 19.6107) (-27.0006, 19.6107) knots 0 0 0 0 1 1 1 1
  line L58 (-28.6096, 18.8906) -> (-27.8899, 19.6107) construction
  line L59 (-27.8899, 19.6107) -> (-27.0006, 19.6107) construction
  line L60 (-26.1114, 16.3897) -> (-27.0006, 16.3897) construction
  spline S10 degree 3 poles (-25.3917, 18.0009) (-25.3917, 17.1112) (-26.1114, 16.3897) (-27.0006, 16.3897) knots 0 0 0 0 1 1 1 1
  line L61 (-25.3917, 18.0009) -> (-25.3917, 17.1112) construction
  line L62 (-25.3917, 17.1112) -> (-26.1114, 16.3897) construction
  line L63 (-27.0006, 19.6107) -> (-26.1114, 19.6107) construction
  spline S11 degree 3 poles (-27.0006, 19.6107) (-26.1114, 19.6107) (-25.3917, 18.8906) (-25.3917, 18.0009) knots 0 0 0 0 1 1 1 1
  line L64 (-26.1114, 19.6107) -> (-25.3917, 18.8906) construction
  line L65 (-25.3917, 18.8906) -> (-25.3917, 18.0009) construction
  line L66 (-24.4006, 15.9224) -> (-30.1006, 19.2133)
  line L67 (-29.6006, 20.0794) -> (-24.4006, 15.9224) construction
  circle A15 centre (-27.0006, 18.0009) radius 2.5
  line L68 (-29.6006, 20.0794) -> (-23.9006, 16.7885)
  line L69 (-24.1506, 16.3554) -> (-27.0006, 18.0009)
  line L70 (-27.0006, 21.2918) -> (-24.1506, 19.6463)
  line L71 (-24.1506, 19.6463) -> (-24.1506, 16.3554)
  line L72 (-27.0006, 18.0009) -> (-29.8506, 18.0009)
  circle A16 centre (-27.0006, 21.0031) radius 0.5
  line L73 (-29.8506, 19.6463) -> (-27.0006, 21.2918)
  circle A17 centre (-29.6006, 16.4998) radius 0.5
  line L74 (-27.0006, 14.71) -> (-29.8506, 16.3554)
  circle A18 centre (-29.6006, 19.502) radius 0.5
  line L75 (-30.1006, 19.2133) -> (-29.6006, 20.0794)
  line L76 (-29.8506, 16.3554) -> (-29.8506, 19.6463)
  line L77 (-23.9006, 16.7885) -> (-30.1006, 19.2133) construction
  circle A19 centre (-27.0006, 14.9987) radius 0.5
  line L78 (-24.6506, 16.0668) -> (-24.1506, 16.9328)
  line L79 (-24.1506, 16.3554) -> (-27.0006, 14.71)
  circle A20 centre (-24.4006, 16.4998) radius 0.5
  line L80 (-23.9006, 16.7885) -> (-24.4006, 15.9224)
  line L81 (-48.0086, 16.3897) -> (-48.8979, 16.3897) construction
  spline S12 degree 3 poles (-48.0086, 16.3897) (-48.8979, 16.3897) (-49.6176, 17.1112) (-49.6176, 18.0009) knots 0 0 0 0 1 1 1 1
  line L82 (-48.8979, 16.3897) -> (-49.6176, 17.1112) construction
  line L83 (-49.6176, 17.1112) -> (-49.6176, 18.0009) construction
  circle A21 centre (-45.4086, 19.502) radius 0.5
  line L84 (-49.6176, 18.0009) -> (-49.6176, 18.8906) construction
  spline S13 degree 3 poles (-49.6176, 18.0009) (-49.6176, 18.8906) (-48.8979, 19.6107) (-48.0086, 19.6107) knots 0 0 0 0 1 1 1 1
  line L85 (-49.6176, 18.8906) -> (-48.8979, 19.6107) construction
  line L86 (-48.8979, 19.6107) -> (-48.0086, 19.6107) construction
  line L87 (-47.1193, 16.3897) -> (-48.0086, 16.3897) construction
  spline S14 degree 3 poles (-46.3996, 18.0009) (-46.3996, 17.1112) (-47.1193, 16.3897) (-48.0086, 16.3897) knots 0 0 0 0 1 1 1 1
  line L88 (-46.3996, 18.0009) -> (-46.3996, 17.1112) construction
  line L89 (-46.3996, 17.1112) -> (-47.1193, 16.3897) construction
  line L90 (-48.0086, 19.6107) -> (-47.1193, 19.6107) construction
  spline S15 degree 3 poles (-48.0086, 19.6107) (-47.1193, 19.6107) (-46.3996, 18.8906) (-46.3996, 18.0009) knots 0 0 0 0 1 1 1 1
  line L91 (-47.1193, 19.6107) -> (-46.3996, 18.8906) construction
  line L92 (-46.3996, 18.8906) -> (-46.3996, 18.0009) construction
  line L93 (-45.4086, 15.9224) -> (-51.1086, 19.2133)
  line L94 (-50.6086, 20.0794) -> (-45.4086, 15.9224) construction
  circle A22 centre (-48.0086, 18.0009) radius 2.5
  line L95 (-50.6086, 20.0794) -> (-44.9086, 16.7885)
  line L96 (-45.1586, 16.3554) -> (-48.0086, 18.0009)
  line L97 (-48.0086, 21.2918) -> (-45.1586, 19.6463)
  line L98 (-45.1586, 19.6463) -> (-45.1586, 16.3554)
  line L99 (-48.0086, 18.0009) -> (-50.8586, 18.0009)
  circle A23 centre (-48.0086, 21.0031) radius 0.5
  line L100 (-50.8586, 19.6463) -> (-48.0086, 21.2918)
  circle A24 centre (-50.6086, 16.4998) radius 0.5
  line L101 (-48.0086, 14.71) -> (-50.8586, 16.3554)
  circle A25 centre (-50.6086, 19.502) radius 0.5
  line L102 (-51.1086, 19.2133) -> (-50.6086, 20.0794)
  line L103 (-50.8586, 16.3554) -> (-50.8586, 19.6463)
  line L104 (-44.9086, 16.7885) -> (-51.1086, 19.2133) construction
  circle A26 centre (-48.0086, 14.9987) radius 0.5
  line L105 (-45.6586, 16.0668) -> (-45.1586, 16.9328)
  line L106 (-45.1586, 16.3554) -> (-48.0086, 14.71)
  circle A27 centre (-45.4086, 16.4998) radius 0.5
  line L107 (-44.9086, 16.7885) -> (-45.4086, 15.9224)
  line L108 (-51.9904, 48.4097) -> (-52.8797, 48.4097) construction
  spline S16 degree 3 poles (-51.9904, 48.4097) (-52.8797, 48.4097) (-53.5994, 49.1311) (-53.5994, 50.0209) knots 0 0 0 0 1 1 1 1
  line L109 (-52.8797, 48.4097) -> (-53.5994, 49.1311) construction
  line L110 (-53.5994, 49.1311) -> (-53.5994, 50.0209) construction
  circle A28 centre (-49.3904, 51.522) radius 0.5
  line L111 (-53.5994, 50.0209) -> (-53.5994, 50.9106) construction
  spline S17 degree 3 poles (-53.5994, 50.0209) (-53.5994, 50.9106) (-52.8797, 51.6306) (-51.9904, 51.6306) knots 0 0 0 0 1 1 1 1
  line L112 (-53.5994, 50.9106) -> (-52.8797, 51.6306) construction
  line L113 (-52.8797, 51.6306) -> (-51.9904, 51.6306) construction
  line L114 (-51.1011, 48.4097) -> (-51.9904, 48.4097) construction
  spline S18 degree 3 poles (-50.3814, 50.0209) (-50.3814, 49.1311) (-51.1011, 48.4097) (-51.9904, 48.4097) knots 0 0 0 0 1 1 1 1
  line L115 (-50.3814, 50.0209) -> (-50.3814, 49.1311) construction
  line L116 (-50.3814, 49.1311) -> (-51.1011, 48.4097) construction
  line L117 (-51.9904, 51.6306) -> (-51.1011, 51.6306) construction
  spline S19 degree 3 poles (-51.9904, 51.6306) (-51.1011, 51.6306) (-50.3814, 50.9106) (-50.3814, 50.0209) knots 0 0 0 0 1 1 1 1
  line L118 (-51.1011, 51.6306) -> (-50.3814, 50.9106) construction
  line L119 (-50.3814, 50.9106) -> (-50.3814, 50.0209) construction
  line L120 (-49.3904, 47.9424) -> (-55.0904, 51.2333)
  line L121 (-54.5904, 52.0993) -> (-49.3904, 47.9424) construction
  circle A29 centre (-51.9904, 50.0209) radius 2.5
  line L122 (-54.5904, 52.0993) -> (-48.8904, 48.8084)
  line L123 (-49.1404, 48.3754) -> (-51.9904, 50.0209)
  line L124 (-51.9904, 53.3118) -> (-49.1404, 51.6663)
  line L125 (-49.1404, 51.6663) -> (-49.1404, 48.3754)
  line L126 (-51.9904, 50.0209) -> (-54.8404, 50.0209)
  circle A30 centre (-51.9904, 53.0231) radius 0.5
  line L127 (-54.8404, 51.6663) -> (-51.9904, 53.3118)
  circle A31 centre (-54.5904, 48.5197) radius 0.5
  line L128 (-51.9904, 46.73) -> (-54.8404, 48.3754)
  circle A32 centre (-54.5904, 51.522) radius 0.5
  line L129 (-55.0904, 51.2333) -> (-54.5904, 52.0993)
  line L130 (-54.8404, 48.3754) -> (-54.8404, 51.6663)
  line L131 (-48.8904, 48.8084) -> (-55.0904, 51.2333) construction
  circle A33 centre (-51.9904, 47.0186) radius 0.5
  line L132 (-49.6404, 48.0867) -> (-49.1404, 48.9528)
  line L133 (-49.1404, 48.3754) -> (-51.9904, 46.73)
  circle A34 centre (-49.3904, 48.5197) radius 0.5
  line L134 (-48.8904, 48.8084) -> (-49.3904, 47.9424)
  point P0 (0, 0)
  point P1 (53.367, 51.955)
  point P2 (48.167, 51.089)
  point P3 (48.667, 48.0867)
  point P4 (51.517, 47.0186)
  point P5 (50.517, 53.0231)
  point P6 (18.997, 18.0009)
  point P7 (-51.9904, 50.0209)
  point P8 (21.3083, 19.974)
  point P9 (18.4583, 21.0421)
  point P10 (16.6083, 16.1058)
  point P11 (16.1083, 19.108)
  point P12 (19.4583, 15.0377)
  point P13 (-24.6506, 19.935)
  point P14 (-27.5006, 21.0031)
  point P15 (-29.3506, 16.0668)
  point P16 (-29.8506, 19.069)
  point P17 (-26.5006, 14.9987)
  point P18 (-45.6586, 19.935)
  point P19 (-48.5086, 21.0031)
  point P20 (-50.3586, 16.0668)
  point P21 (-50.8586, 19.069)
  point P22 (-47.5086, 14.9987)
  point P23 (-49.6404, 51.955)
  point P24 (-52.4904, 53.0231)
  point P25 (-54.3404, 48.0867)
  point P26 (-54.8404, 51.089)
  point P27 (-51.4904, 47.0186)
  dimension "d51" = 2.85
  dimension "d52" = 1
  dimension "d53" = 360
  dimension "d54" = 5
  dimension "d112" = 2.85
  dimension "d113" = 1
  dimension "d114" = 360
  dimension "d115" = 5
  dimension "d120" = 2.85
  dimension "d121" = 1
  dimension "d122" = 360
  dimension "d123" = 5
  dimension "d130" = 2.85
  dimension "d131" = 1
  dimension "d132" = 360
  dimension "d133" = 5
  dimension "d142" = 2.85
  dimension "d143" = 1
  dimension "d144" = 360
  dimension "d145" = 5
  constraints: 150 end point, 25 coincident, 25 point on line, 20 midpoint, 10 horizontal alignment, 10 parallel, 5 centre point, 5 horizontal, 5 perpendicular, 300 other
  measures "d51" distance of L6.start L6.end
  measures "d52" distance of L15.end L13.start
  measures "d54" diameter of A1
  measures "d112" distance of L45.start L45.end
  measures "d113" distance of L50.start L40.end
  measures "d115" diameter of A8
  measures "d120" distance of L72.start L72.end
  measures "d121" distance of L77.start L67.end
  measures "d123" diameter of A15
  measures "d130" distance of L99.start L99.end
  measures "d131" distance of L104.start L94.end
  measures "d133" diameter of A22
  measures "d142" distance of L126.start L126.end
  measures "d143" distance of L131.start L121.end
  measures "d145" diameter of A29
sketch "magnets" plane through (0, 0, 0) normal (0, 1, 0) x (-1, 0, 0)
  circle A0 centre (41.0211, 40.025) radius 2.7
  line L0 (0, -67.9804) -> (0, 68.0217) projected
  line L1 (76.0481, 0) -> (-83.6298, 0) projected
  circle A1 centre (41.0211, 30.025) radius 2.7
  circle A2 centre (31.0211, 40.025) radius 2.7
  circle A3 centre (31.0211, 30.025) radius 2.7
  circle A4 centre (-31.9986, 40.025) radius 2.7
  circle A5 centre (-31.9986, 30.025) radius 2.7
  circle A6 centre (-41.9986, 40.025) radius 2.7
  circle A7 centre (-41.9986, 30.025) radius 2.7
  circle A8 centre (-53.9813, 4.9979) radius 2.7
  circle A9 centre (-53.9813, -5.0021) radius 2.7
  circle A10 centre (-63.9813, 4.9979) radius 2.7
  circle A11 centre (-63.9813, -5.0021) radius 2.7
  circle A12 centre (41.0211, -40.025) radius 2.7
  circle A13 centre (41.0211, -30.025) radius 2.7
  circle A14 centre (31.0211, -40.025) radius 2.7
  circle A15 centre (31.0211, -30.025) radius 2.7
  circle A16 centre (-31.9986, -40.025) radius 2.7
  circle A17 centre (-31.9986, -30.025) radius 2.7
  circle A18 centre (-41.9986, -40.025) radius 2.7
  circle A19 centre (-41.9986, -30.025) radius 2.7
  point P0 (0, 0)
  point P1 (-31.9986, 40.025)
  point P2 (-53.9813, 4.9979)
  point P3 (-31.9986, -40.025)
  dimension "d6" = 5.4
  dimension "d9" = 10
  dimension "d12" = 10
  dimension "d19" = 5.4
  dimension "d20" = 10
  dimension "d21" = 10
  dimension "d26" = 5.4
  dimension "d27" = 10
  dimension "d28" = 10
  constraints: 20 centre point, 10 symmetric about line, 2 coincident, 1 horizontal, 1 vertical, 14 other
  measures "d6" diameter of A0
  measures "d9" distance of A0.centre A1.centre
  measures "d12" distance of A0.centre A2.centre
  measures "d19" diameter of A4
  measures "d20" distance of A4.centre A5.centre
  measures "d21" distance of A4.centre A6.centre
  measures "d26" diameter of A8
  measures "d27" distance of A8.centre A9.centre
  measures "d28" distance of A8.centre A10.centre
sketch "base" plane through (0, 0, 0) normal (0, 1, 0) x (-1, 0, 0)
  line L0 (56, 57) -> (-66, 57)
  line L1 (-66, 57) -> (-66, 0)
  line L2 (-66, 0) -> (56, 0)
  line L3 (56, 0) -> (56, 57)
  line L4 (25.0111, 50.0209) -> (25.0111, 68.0217) projected
  line L5 (6.5015, 50.0209) -> (25.0111, 50.0209) projected
  line L6 (-25.0111, 50.0209) -> (-6.5015, 50.0209) projected
  line L7 (-25.0111, 50.0209) -> (-25.0111, 68.0217) projected
  line L8 (25.0111, 50.0209) -> (-25.0111, 50.0209)
  line L9 (-25.0111, 50.0209) -> (-25.0111, 68.0217)
  line L10 (-25.0111, 68.0217) -> (25.0111, 68.0217)
  line L11 (25.0111, 68.0217) -> (25.0111, 50.0209)
  line L12 (25.0111, 57) -> (25.0111, 50.0209)
  line L13 (-25.0111, 50.0209) -> (-25.0111, 57)
  line L14 (14.5, 0) -> (5.5, 0)
  line L15 (14, 50.0209) -> (-14, 50.0209)
  line L16 (-4.9766, 0.0207) -> (-4.9766, 0)
  line L17 (-22.9775, 0.0207) -> (-22.9775, 0)
  point P0 (0, 0)
  point P1 (0, 0)
  point P2 (51.017, 50.0209)
  point P3 (18.997, 18.0009)
  point P4 (9.0011, 44.0068)
  point P5 (-8.9998, 44.0068)
  point P6 (-27.0006, 18.0009)
  point P7 (-48.0086, 18.0009)
  point P8 (-51.9904, 50.0209)
  point P9 (-22.9775, 13.5103)
  dimension "d29" = 56
  dimension "d30" = 66
  dimension "d31" = 57
  constraints: 28 end point, 8 point on line, 4 horizontal, 4 parallel, 4 perpendicular, 1 collinear
  measures "d29" distance from line of point (0, 0) L3
  measures "d30" distance from line of point (0, 0) L1
  measures "d31" distance from line of point (0, 0) L0
extrude "Extrusion1" add sketch "base" against normal blind 7 contours L3 L2 L1 L0 L7 L6 L8 L5 L4
extrude "Extrusion2" cut sketch "magnets" against normal blind 2.2 contours A0 | A1 | A2 | A3 | A4 | A5 | A6 | A7 | A8 | A10
sketch "Sketch8" plane through (0, 0, 0) normal (0, 1, 0) x (1, 0, 0)
  line L0 (-51.017, -53.3118) -> (-53.867, -51.6663)
  line L1 (-53.867, -51.6663) -> (-53.867, -48.3754)
  line L2 (-53.867, -48.3754) -> (-51.017, -46.73)
  line L3 (-51.017, -46.73) -> (-48.167, -48.3754)
  line L4 (-48.167, -48.3754) -> (-48.167, -51.6663)
  line L5 (-48.167, -51.6663) -> (-51.017, -53.3118)
  circle A0 centre (-51.017, -53.0231) radius 0.5
  circle A1 centre (-53.617, -51.522) radius 0.5
  circle A2 centre (-53.617, -48.5197) radius 0.5
  circle A3 centre (-51.017, -47.0186) radius 0.5
  circle A4 centre (-48.417, -48.5197) radius 0.5
  circle A5 centre (-48.417, -51.522) radius 0.5
  line L6 (-18.997, -21.2918) -> (-21.847, -19.6463)
  line L7 (-21.847, -19.6463) -> (-21.847, -16.3554)
  line L8 (-21.847, -16.3554) -> (-18.997, -14.71)
  line L9 (-18.997, -14.71) -> (-16.147, -16.3554)
  line L10 (-16.147, -16.3554) -> (-16.147, -19.6463)
  line L11 (-16.147, -19.6463) -> (-18.997, -21.2918)
  circle A6 centre (-18.997, -21.0031) radius 0.5
  circle A7 centre (-21.597, -19.502) radius 0.5
  circle A8 centre (-21.597, -16.4998) radius 0.5
  circle A9 centre (-18.997, -14.9987) radius 0.5
  circle A10 centre (-16.397, -16.4998) radius 0.5
  circle A11 centre (-16.397, -19.502) radius 0.5
  line L12 (27.0006, -21.2918) -> (24.1506, -19.6463)
  line L13 (24.1506, -19.6463) -> (24.1506, -16.3554)
  line L14 (24.1506, -16.3554) -> (27.0006, -14.71)
  line L15 (27.0006, -14.71) -> (29.8506, -16.3554)
  line L16 (29.8506, -16.3554) -> (29.8506, -19.6463)
  line L17 (29.8506, -19.6463) -> (27.0006, -21.2918)
  circle A12 centre (27.0006, -21.0031) radius 0.5
  circle A13 centre (24.4006, -19.502) radius 0.5
  circle A14 centre (24.4006, -16.4998) radius 0.5
  circle A15 centre (27.0006, -14.9987) radius 0.5
  circle A16 centre (29.6006, -16.4998) radius 0.5
  circle A17 centre (29.6006, -19.502) radius 0.5
  line L18 (48.0086, -21.2918) -> (45.1586, -19.6463)
  line L19 (45.1586, -19.6463) -> (45.1586, -16.3554)
  line L20 (45.1586, -16.3554) -> (48.0086, -14.71)
  line L21 (48.0086, -14.71) -> (50.8586, -16.3554)
  line L22 (50.8586, -16.3554) -> (50.8586, -19.6463)
  line L23 (50.8586, -19.6463) -> (48.0086, -21.2918)
  circle A18 centre (48.0086, -21.0031) radius 0.5
  circle A19 centre (45.4086, -19.502) radius 0.5
  circle A20 centre (45.4086, -16.4998) radius 0.5
  circle A21 centre (48.0086, -14.9987) radius 0.5
  circle A22 centre (50.6086, -16.4998) radius 0.5
  circle A23 centre (50.6086, -19.502) radius 0.5
  line L24 (51.9904, -53.3118) -> (49.1404, -51.6663)
  line L25 (49.1404, -51.6663) -> (49.1404, -48.3754)
  line L26 (49.1404, -48.3754) -> (51.9904, -46.73)
  line L27 (51.9904, -46.73) -> (54.8404, -48.3754)
  line L28 (54.8404, -48.3754) -> (54.8404, -51.6663)
  line L29 (54.8404, -51.6663) -> (51.9904, -53.3118)
  circle A24 centre (51.9904, -53.0231) radius 0.5
  circle A25 centre (49.3904, -51.522) radius 0.5
  circle A26 centre (49.3904, -48.5197) radius 0.5
  circle A27 centre (51.9904, -47.0186) radius 0.5
  circle A28 centre (54.5904, -48.5197) radius 0.5
  circle A29 centre (54.5904, -51.522) radius 0.5
  point P0 (0, 0)
  point P1 (-18.997, -18.0009)
  point P2 (27.0006, -18.0009)
  point P3 (48.0086, -18.0009)
  point P4 (51.9904, -50.0209)
  point P5 (-51.017, -50.0209)
  point P6 (-18.997, -18.0009)
  point P7 (27.0006, -18.0009)
  point P8 (48.0086, -18.0009)
  point P9 (51.9904, -50.0209)
  constraints: 60 end point, 30 centre point
extrude "Extrusion4" cut sketch "Sketch8" against normal blind 2.3
hole "Hole2" at (-51.017, 0, 50.0209) at (-18.997, 0, 18.0009) at (27.0006, 0, 18.0009) at (48.0086, 0, 18.0009) at (51.9904, 0, 50.0209) direction (0, -1, 0) diameter 2 end through all counterbore diameter 4 counterbore depth 4.2